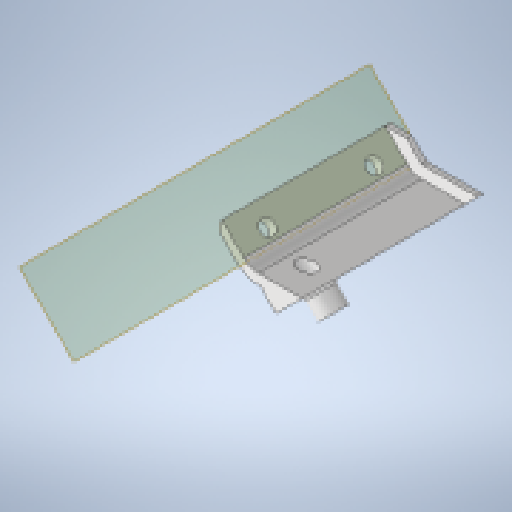
# Autodesk Inventor part: GripperHandleRight
Saved by Autodesk Inventor 2025.1 (Build 291241000, 241)
## iProperties
Created: 2026-05-06
Part Number: GripperHandleRight
Material: Generic
Document SubType Name: Modeling
Designer: User
Density: 1 g/cm^3
Appearance: Default
Author: User
## iProperties of the stored document GripperHandleRight_3DPrint.ipt
Created: 2026-05-06
Part Number: GripperHandleRight_3DPrint
Material: Generic
Document SubType Name: Modeling
Designer: User
Density: 1 g/cm^3
Appearance: Default
Author: User
Autodesk Inventor part; units mm, degrees
ref_plane "YZ Plane" through (0, 0, 0) normal (1, 0, 0) x (0, 1, 0)
ref_plane "XZ Plane" through (0, 0, 0) normal (0, 1, 0) x (-1, 0, 0)
ref_plane "XY Plane" through (0, 0, 0) normal (0, 0, 1) x (1, 0, 0)
ref_plane "Work Plane1" through (-26.7198, -9.0991, 72.4417) normal (-0.7071068, -0.7071068, 0) x (0.7071068, -0.7071068, 0)
sketch "Sketch1" plane through (-26.7198, -9.0991, 72.4417) normal (-0.7071068, -0.7071068, 0) x (0.7071068, -0.7071068, 0)
  line L0 (-1.6569, 2.5) -> (-1.6569, -60.4376) projected
  line L1 (-15.5563, 2.5) -> (-1.6569, 2.5) projected
  line L2 (-15.5563, 2.5) -> (-15.5563, 0) projected
  line L3 (-7.7782, 0) -> (-15.5563, 0) projected
  line L4 (-7.7782, -60.4376) -> (-7.7782, 0) projected
  line L5 (-7.7782, -60.4376) -> (-1.6569, -60.4376) projected
  circle A0 centre (58.298, -34.4266) radius 35
  line L6 (58.298, -34.4266) -> (-7.7782, -34.4266)
  line L7 (58.298, -34.4266) -> (124.3741, -34.4266) construction
  line L8 (-7.7782, -28.4266) -> (58.298, -28.4266)
  line L9 (58.298, -28.4266) -> (124.3741, -28.4266)
  point P0 (12.4597, -72.4417)
  point P1 (-1.6569, -28.4266)
  point P2 (-7.7782, -28.4266)
  dimension "d0" = 180
  dimension "d1" = 6
  constraints: 8 end point, 1 centre point, 1 collinear, 1 horizontal, 1 point on line, 3 other
  measures "d0" angle of L6 L7
  measures "d1" distance between parallel lines of L6 L8
extrude "Extrusion1" add sketch "Sketch1" along normal blind 2 contours L0 L6 L4 L8 | L0 L5 L4 L6
sketch "Sketch2" plane through (-27.8914, -7.9275, 12.0041) normal (0, 0, -1) x (-0.7071068, -0.7071068, 0)
  line L0 (0, 6.1213) -> (0, 0) projected
  line L1 (0, 0) -> (2, 0) projected
  line L2 (2, 6.1213) -> (2, 0) projected
  line L3 (0, 6.1213) -> (2, 6.1213) projected
  point P0 (-25.3278, -14.1166)
extrude "Extrusion2" add sketch "Sketch2" along normal blind 0.2
sketch "Sketch3" plane through (-27.8914, -7.9275, 11.8041) normal (0, 0, -1) x (-0.7071068, 0.7071068, 0)
  arc A0 (-2.8284, 1.1716) -> (0, 0) centre (0, 4) ccw projected
  line L0 (6.1213, 0) -> (0, 0) projected
  line L1 (-2.8284, 1.1716) -> (-54.1742, 52.5173) projected
  line L2 (0, -2) -> (6.1213, -2) projected
  line L3 (0, 0) -> (0, -2) projected
  line L4 (-55.5884, 51.1031) -> (-4.2426, -0.2426)
  arc A1 (-4.2426, -0.2426) -> (0, -2) centre (0, 4) ccw
  line L5 (-9.2664, 7.2928) -> (-12.0609, 7.2928) projected
  line L6 (-9.2664, 7.2928) -> (5.6067, 7.2928) projected
  line L7 (-12.5609, 16.1266) -> (-12.5609, 10.1266) projected
  line L8 (-8.9496, 7.2928) -> (-8.9496, 0)
  line L9 (-8.9496, 7.2928) -> (-1.6569, 7.2928) construction
  line L10 (-8.9496, 0) -> (-4.4721, 0)
  line L11 (-8.9496, 0) -> (-4.4721, 0) construction
  point P0 (-14.1166, 25.3278)
  point P1 (-4.4853, 0)
  dimension "d6" = 2
  dimension "d7" = 90
  dimension "d8" = 0
  constraints: 10 end point, 3 point on circle, 2 equal length, 2 horizontal, 2 point on line, 1 centre point, 1 other
  measures "d6" distance between parallel lines of L1 L4
  measures "d7" angle of L8 L9
  measures "d8" distance between parallel lines of L10 L11
extrude "Extrusion3" add sketch "Sketch3" against normal up to surface (32.211 mm away) contours A0 L3 A1 L4 L8 L1 | L4 L10 L8
sketch "Sketch4" plane through (-27.8914, -7.9275, 11.8041) normal (0, 0, -1) x (-0.7071068, 0.7071068, 0)
  line L0 (6.1213, 0) -> (0, 0) projected
  arc A0 (-2.8284, 1.1716) -> (0, 0) centre (0, 4) ccw projected
  line L1 (-2.8284, 1.1716) -> (-8.9496, 7.2928) projected
  line L2 (-8.9496, 7.2928) -> (-8.9496, 0) projected
  line L3 (-8.9496, 0) -> (-4.4853, 0) projected
  line L4 (-4.4853, 0) -> (-4.2426, -0.2426) projected
  arc A1 (-4.2426, -0.2426) -> (0, -2) centre (0, 4) ccw projected
  line L5 (0, -2) -> (6.1213, -2) projected
  line L6 (6.1213, -2) -> (6.1213, 0) projected
  line L7 (3.1213, 3) -> (6.1213, 0) projected
  line L8 (-1.1213, 3) -> (3.1213, 3) projected
  line L9 (-18.8648, 20.7435) -> (-1.1213, 3) projected
  line L10 (-8.9496, 7.2928) -> (-8.9496, 10.8283)
  point P0 (-14.1166, 25.3278)
  constraints: 2 end point, 1 point on line, 1 vertical
extrude "Extrusion4" add sketch "Sketch4" along normal blind 1
fillet "Fillet1" radius 2 1 edges at (-33.634, -5.0133, 27.4096)
sketch "Sketch5" plane through (-21.563, -14.2558, 44.0151) normal (0.7071068, -0.7071068, 0) x (-0.7071068, -0.7071068, 0)
  circle A0 centre (-3.6464, 6) radius 2.5 projected
  point P0 (-25.3278, 44.0151)
extrude "Extrusion5" add sketch "Sketch5" along normal blind 4
chamfer "Chamfer1" distance 0.5 angle 45 1 edges at (-17.2169, -9.9097, 38.0151)
sketch "Sketch6" plane through (-16.1562, -14.5059, 38.0151) normal (0.7071068, -0.7071068, 0) x (-0.7071068, -0.7071068, 0)
  circle A0 centre (0, 0) radius 1.5 projected
  point P0 (-21.6814, 38.0151)
extrude "Extrusion6" cut sketch "Sketch6" against normal through all
sketch "Sketch7" plane through (-28.134, -10.5133, 72.4417) normal (-0.7071068, -0.7071068, 0) x (0, 0, 1)
  line L0 (-61.6376, 5.7782) -> (-28.4266, 5.7782) projected
  line L1 (-61.6376, 1.6569) -> (-61.6376, 5.7782) projected
  line L2 (-28.4266, 1.6569) -> (-61.6376, 1.6569) projected
  line L3 (-28.4266, 1.6569) -> (-28.4266, 5.7782) projected
  line L4 (-28.4266, 7.7782) -> (-28.4266, 5.7782) projected
  line L5 (-28.4266, 5.7782) -> (-32.4266, 5.7782)
  line L6 (-32.4266, 5.7782) -> (-32.4266, 1.6569)
  line L7 (-32.4266, 1.6569) -> (-28.4266, 1.6569)
  line L8 (-28.4266, 1.6569) -> (-28.4266, 5.7782)
  circle A0 centre (-34.4873, 3.7175) radius 2.0607
  circle A1 centre (-34.4873, 3.7175) radius 1.5
  point P0 (-72.4417, -12.4597)
  dimension "d21" = 4
  dimension "d22" = 3
  constraints: 8 end point, 3 tangent, 2 centre point, 2 parallel, 1 coincident, 1 horizontal, 1 perpendicular, 1 point on line
  measures "d21" distance of L7.end L6.end
  measures "d22" diameter of A1
extrude "Extrusion7" cut sketch "Sketch7" against normal blind 10 contours A1
sketch "Sketch8" plane through (-28.134, -10.5133, 72.4417) normal (-0.7071068, -0.7071068, 0) x (0, 0, 1)
  circle A0 centre (-34.4873, 3.7175) radius 1.5 projected
  line L0 (-61.6376, 5.7782) -> (-28.4266, 5.7782) projected
  line L1 (-61.6376, 1.6569) -> (-61.6376, 5.7782) projected
  line L2 (-28.4266, 1.6569) -> (-61.6376, 1.6569) projected
  line L3 (-28.4266, 1.6569) -> (-28.4266, 5.7782) projected
  line L4 (-61.6376, 5.7782) -> (-57.6376, 5.7782)
  line L5 (-57.6376, 5.7782) -> (-57.6376, 1.6569)
  line L6 (-57.6376, 1.6569) -> (-61.6376, 1.6569)
  line L7 (-61.6376, 1.6569) -> (-61.6376, 5.7782)
  circle A1 centre (-55.577, 3.7175) radius 2.0607
  circle A2 centre (-55.577, 3.7175) radius 1.5
  point P0 (-72.4417, -12.4597)
  dimension "d25" = 4
  dimension "d26" = 3
  constraints: 8 end point, 3 tangent, 2 centre point, 2 parallel, 1 coincident, 1 horizontal, 1 perpendicular, 1 point on line
  measures "d25" distance of L5.end L6.end
  measures "d26" diameter of A2
extrude "Extrusion8" cut sketch "Sketch8" against normal blind 10 contours A2
body "Solid1"
